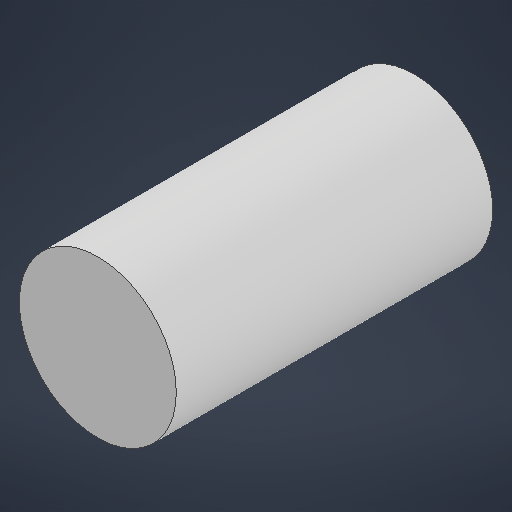
# Autodesk Inventor part: rim-v1
Saved by Autodesk Inventor 2026.2 (Build 302298010, 298A)
## iProperties
Created: 2026-05-11
Part Number: rim-v1
Material: Generic
Document SubType Name: Modeling
Designer: karol
Density: 1 g/cm^3
Appearance: Default
Author: karol
Autodesk Inventor part; units mm, degrees
ref_plane "YZ Plane" through (0, 0, 0) normal (1, 0, 0) x (0, 1, 0)
ref_plane "XZ Plane" through (0, 0, 0) normal (0, 1, 0) x (-1, 0, 0)
ref_plane "XY Plane" through (0, 0, 0) normal (0, 0, 1) x (1, 0, 0)
ref_plane "Work Plane1" through (0, 0, 0.5) normal (0, 0, 1) x (1, 0, 0)
sketch "Sketch1" plane through (0, 0, 0.5) normal (0, 0, 1) x (1, 0, 0)
  arc A0 (13, 1.882) -> (13, 4.118) centre (14, 3) ccw projected
  arc A1 (13, 1.882) -> (13, 4.118) centre (14, 3) ccw projected
  line L0 (13, 4.118) -> (13, 1.882) projected
  circle A2 centre (14, 3) radius 6
  circle A3 centre (14, 3) radius 4
  circle A4 centre (14, 3) radius 1.7
  line L1 (12.7, 1.9046) -> (12.7, 4.0954)
  point P0 (0, 0)
  dimension "d0" = 12
  dimension "d1" = 8
  dimension "d2" = 0.2
  dimension "d3" = 0.3
  constraints: 3 centre point, 3 coincident, 2 end point, 2 point on circle, 1 parallel, 1 vertical
  measures "d0" diameter of A2
  measures "d1" diameter of A3
  measures "d2" radial gap between concentric circles of A0 A4
  measures "d3" distance between parallel lines of L0 L1
extrude "Extrusion1" add sketch "Sketch1" along normal blind 21.5 contours A3 | L1 A4 picked at (12.5667, 3)
ref_plane "Work Plane2" through (14, 3, 18) normal (0, 0, 1) x (1, 0, 0)
sketch "Sketch2" plane through (14, 3, 18) normal (0, 0, 1) x (1, 0, 0)
  circle A0 centre (0, 0) radius 4 projected
  arc A1 (-1.3, -1.0954) -> (-1.3, 1.0954) centre (0, 0) ccw projected
  line L0 (-1.3, -1.0954) -> (-1.3, 1.0954) projected
  circle A2 centre (0, 0) radius 3
  point P0 (-14, -3)
  dimension "d7" = 6
  constraints: 1 centre point, 1 coincident
  measures "d7" diameter of A2
extrude "Extrusion2" cut sketch "Sketch2" against normal blind 2 contours A0
ref_plane "Work Plane3" through (9.7, 1.9046, 0.5) normal (1, 0, 0) x (0, 0, -1)
sketch "Sketch3" plane through (9.7, 1.9046, 0.5) normal (1, 0, 0) x (0, 0, -1)
  circle A0 centre (-2.5, 1) radius 0.8
  line L0 (-21.5, 0) -> (-21.5, 2.1909) projected
  point P0 (0.5, -1.9046)
  dimension "d11" = 1.6
  dimension "d12" = 1
  dimension "d15" = 19
  constraints: 1 centre point
  measures "d11" diameter of A0
  measures "d12" vertical distance of L0.start A0.centre
  measures "d15" distance from line of L0 A0.centre
extrude "Extrusion3" cut sketch "Sketch3" along normal blind 3.1
chamfer "Chamfer1" distance 0.25 angle 45 1 edges at (10.0014, 2.8949, 3.7999)
ref_plane "Work Plane4" through (14, 3, 13) normal (0, 0, 1) x (1, 0, 0)
sketch "Sketch4" plane through (14, 3, 13) normal (0, 0, 1) x (1, 0, 0)
  circle A0 centre (0, 0) radius 4 projected
  circle A1 centre (0, 0) radius 4 projected
  circle A2 centre (0, 0) radius 3 projected
  point P0 (-14, -3)
extrude "Extrusion4" cut sketch "Sketch4" against normal blind 2
sketch "Sketch6" plane through (14, 3, 22) normal (0, 0, 1) x (1, 0, 0)
  circle A0 centre (0, 0) radius 3 projected
  circle A1 centre (0, 0) radius 6
  circle A2 centre (0, 0) radius 6.4
  point P0 (-14, -3)
  dimension "d22" = 12
  dimension "d23" = 12.8
  constraints: 2 centre point, 2 coincident
  measures "d22" diameter of A1
  measures "d23" diameter of A2
extrude "Extrusion5" add sketch "Sketch6" against normal blind 25 contours A2
extrude "Extrusion6" add sketch "Sketch6" along normal blind 0.8 contours A0 | A1 | A2
ref_plane "Płaszczyzna konstrukcyjna5" through (7.6, 1.9046, 0.5) normal (1, 0, 0) x (0, 0, -1)
sketch "Szkic7" plane through (7.6, 1.9046, 0.5) normal (1, 0, 0) x (0, 0, -1)
  spline S0 degree 8 poles (-1.7, 1) (-1.7, 1.091) (-1.7118, 1.1817) (-1.7354, 1.2697) (-1.7694, 1.3549) (-1.8161, 1.4346) (-1.8691, 1.5053) (-1.931, 1.5692) (-2.0525, 1.6666) (-2.1094, 1.7038) (-2.1697, 1.7354) (-2.2328, 1.761) (-2.2981, 1.7804) (-2.3649, 1.7935) (-2.4325, 1.8) (-2.5948, 1.8) (-2.6895, 1.7872) (-2.7823, 1.7614) (-2.8709, 1.7235) (-2.9537, 1.6737) (-3.0292, 1.6129) (-3.0952, 1.5431) (-3.1865, 1.4152) (-3.2179, 1.3621) (-3.2446, 1.3061) (-3.2664, 1.2478) (-3.283, 1.1876) (-3.2942, 1.1261) (-3.2999, 1.0636) (-3.3002, 0.9153) (-3.2897, 0.8293) (-3.2688, 0.7454) (-3.2379, 0.6648) (-3.1973, 0.5884) (-3.148, 0.5177) (-3.091, 0.4543) (-2.9736, 0.3512) (-2.9147, 0.3094) (-2.8516, 0.2737) (-2.785, 0.2445) (-2.7155, 0.2223) (-2.6443, 0.2074) (-2.5722, 0.2) (-2.4272, 0.2) (-2.3545, 0.2075) (-2.2826, 0.2227) (-2.2127, 0.2453) (-2.1455, 0.2749) (-2.082, 0.3112) (-2.0229, 0.3537) (-1.9062, 0.4575) (-1.8501, 0.5206) (-1.8015, 0.5907) (-1.7616, 0.6665) (-1.7311, 0.7466) (-1.7105, 0.8296) (-1.7, 0.9143) (-1.7, 1) knots 0 0 0 0 0 0 0 0 0 0.141182 0.141182 0.141182 0.141182 0.141182 0.141182 0.141182 0.250231 0.250231 0.250231 0.250231 0.250231 0.250231 0.250231 0.403315 0.403315 0.403315 0.403315 0.403315 0.403315 0.403315 0.500281 0.500281 0.500281 0.500281 0.500281 0.500281 0.500281 0.634545 0.634545 0.634545 0.634545 0.634545 0.634545 0.634545 0.750288 0.750288 0.750288 0.750288 0.750288 0.750288 0.750288 0.867021 0.867021 0.867021 0.867021 0.867021 0.867021 0.867021 1 1 1 1 1 1 1 1 1 projected
  point P0 (0.5, -1.9046)
  constraints: 2 other
extrude "Wyciągnięcie proste7" cut sketch "Szkic7" along normal blind 1
thread "Gwint1" size "M2x0.4" class "6H" standard "ANSI Metric M Profile" full length
body "Solid1"
